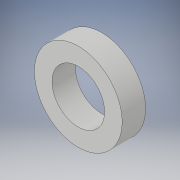
# Autodesk Inventor part: washer
Saved by Autodesk Inventor 2017 (Build 210142000, 142)
## iProperties
Created: 2020-09-15
Part Number: washer
Material: Generic
Document SubType Name: Sheet Metal
Designer: agustin
Density: 1 g/cm^3
Appearance: Default
Sheet Metal Rule: Default
Author: agustin
Autodesk Inventor part; units mm, degrees
ref_plane "YZ Plane" through (0, 0, 0) normal (1, 0, 0) x (0, 1, 0)
ref_plane "XZ Plane" through (0, 0, 0) normal (0, 1, 0) x (-1, 0, 0)
ref_plane "XY Plane" through (0, 0, 0) normal (0, 0, 1) x (1, 0, 0)
sketch "Sketch1" plane through (0, 0, 0) normal (0, 0, 1) x (1, 0, 0)
  circle A0 centre (0, 0) radius 4.5 projected
  circle A1 centre (0, 0) radius 4 projected
  arc A2 (-6.9621, 2.7892) -> (0.4847, -7.4843) centre (0, 0) ccw projected
  circle A3 centre (0, 0) radius 7.5
  point P0 (0, 0)
  constraints: 1 coincident, 3 other
extrude "Extrusion1" add sketch "Sketch1" along normal blind 4 contours A3 A2
scale "Scale1" factors (0.5, 0.5, 0.5) then translate (0, 0, 1) bodies 1
equation "\"BendRadius\" = Thickness"
equation "\"BendReliefWidth\" = Thickness"
equation "\"BendReliefDepth\" = 0.5 * Thickness"
equation "\"CornerReliefSize\" = 4 * Thickness"
equation "\"MinimumRemnant\" = 2 * Thickness"
equation "\"TransitionRadius\" = BendRadius"
equation "\"JacobiRadiusSize\" = Thickness"
equation "\"GapSize\" = Thickness"
equation "\"Thickness\" = 0.5"
body "Solid1"
